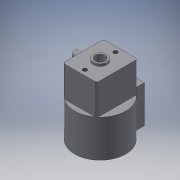
# Autodesk Inventor part: Motor-Body
Saved by Autodesk Inventor 2019 (Build 230136000, 136)
## iProperties
Created: 2021-01-03
Part Number: Motor-Body
Material: Generic
Document SubType Name: Modeling
Designer: Sam
Density: 1 g/cm^3
Appearance: Default
Author: Sam
Autodesk Inventor part; units mm, degrees
ref_plane "YZ Plane" through (0, 0, 0) normal (1, 0, 0) x (0, 1, 0)
ref_plane "XZ Plane" through (0, 0, 0) normal (0, 1, 0) x (-1, 0, 0)
ref_plane "XY Plane" through (0, 0, 0) normal (0, 0, 1) x (1, 0, 0)
sketch "Sketch1" plane through (0, 0, 0) normal (0, 1, 0) x (-1, 0, 0)
  circle A0 centre (0, 0) radius 7.5
  line L0 (-3, -7.5) -> (7, -7.5)
  line L1 (7, -7.5) -> (7, -10)
  line L2 (7, -10) -> (-3, -10)
  line L3 (-3, -10) -> (-3, -7.5)
  circle A1 centre (0, 0) radius 1.5
  dimension "d0" = 15
  dimension "d1" = 3
  dimension "d2" = 10
  dimension "d4" = 10
  dimension "d15" = 3
  constraints: 8 end point, 2 centre point, 2 coincident, 2 parallel, 1 horizontal, 1 perpendicular, 1 tangent
  measures "d0" diameter of A0
  measures "d1" distance from line of point (0, 0) L3
  measures "d2" distance of L1.end L2.end
  measures "d4" distance from line of L2 point (0, 0)
  measures "d15" diameter of A1
extrude "Extrusion3" add sketch "Sketch1" along normal blind 20
sketch "Sketch3" plane through (0, 20, 0) normal (0, 1, 0) x (1, 0, 0)
  line L0 (5, -6) -> (-5, -6)
  line L1 (-5, -6) -> (-5, 6)
  line L2 (-5, 6) -> (5, 6)
  line L3 (5, 6) -> (5, -6)
  line L4 (15, -15) -> (-15, -15)
  line L5 (-15, -15) -> (-15, 15)
  line L6 (-15, 15) -> (15, 15)
  line L7 (15, 15) -> (15, -15)
  point P0 (0, 0)
  point P1 (0, -6)
  point P2 (-5, 0)
  dimension "d18" = 10
  dimension "d19" = 12
  dimension "d20" = 30
  dimension "d21" = 30
  dimension "d22" = 15
  dimension "d23" = 15
  constraints: 16 end point, 4 parallel, 2 horizontal, 2 midpoint, 2 perpendicular, 1 horizontal alignment, 1 vertical alignment
  measures "d18" distance of L0.start L0.end
  measures "d19" distance of L0.end L1.end
  measures "d20" distance of L4.start L4.end
  measures "d21" distance of L6.end L4.start
  measures "d22" distance from line of point (0, 0) L4
  measures "d23" distance from line of point (0, 0) L7
extrude "Extrusion4" cut sketch "Sketch3" against normal blind 9
sketch "Sketch4" plane through (-7, 0, -10) normal (-1, 0, 0) x (0, 0, 1)
  circle A0 centre (1.3, 9.5) radius 1
  circle A1 centre (1.3, 7) radius 1
  circle A2 centre (1.3, 4.5) radius 1
  circle A3 centre (1.3, 2) radius 1
  line L0 (2.5, 0) -> (17.5, 0) projected
  line L1 (0, 0) -> (0, 11) projected
  point P0 (10, 0)
  dimension "d26" = 2
  dimension "d27" = 2.5
  dimension "d28" = 2.5
  dimension "d29" = 2.5
  dimension "d30" = 2
  dimension "d31" = 1.3
  constraints: 4 centre point, 3 equal radius, 3 vertical alignment
  measures "d26" diameter of A0
  measures "d27" distance of A1.centre A0.centre
  measures "d28" distance of A2.centre A1.centre
  measures "d29" distance of A2.centre A3.centre
  measures "d30" distance from line of L0 A3.centre
  measures "d31" distance from line of L1 A3.centre
extrude "Extrusion5" add sketch "Sketch4" along normal blind 9
sketch "Sketch5" plane through (0, 20, 0) normal (0, 1, 0) x (1, 0, 0)
  point P0 (0, 0)
  point P1 (0, -4.5)
  point P2 (0, 4.5)
  dimension "d34" = 9
  dimension "d35" = 4.5
  constraints: 2 vertical alignment
  measures "d34" distance of point (0, 4.5) point (0, -4.5)
  measures "d35" distance of point (0, 0) point (0, -4.5)
hole "Hole1" at (0, 20, 4.5) at (0, 20, -4.5) direction (0, -1, 0) diameter 1.221 depth 5.3 tip angle 118 thread size "M1.6x0.35" class "6H" standard "ISO Metric profile"
sketch "Sketch6" plane through (0, 0, 0) normal (0, -1, 0) x (1, 0, 0)
  circle A0 centre (0, 0) radius 3
  circle A1 centre (0, 0) radius 1.5 projected
  dimension "d43" = 6
  constraints: 1 centre point, 1 coincident
  measures "d43" diameter of A0
extrude "Extrusion6" add sketch "Sketch6" along normal blind 1
sketch "Sketch7" plane through (0, 20, 0) normal (0, 1, 0) x (1, 0, 0)
  circle A0 centre (0, 0) radius 1.5 projected
  circle A1 centre (0, 0) radius 2
  dimension "d46" = 4
  constraints: 1 centre point, 1 coincident
  measures "d46" diameter of A1
extrude "Extrusion7" add sketch "Sketch7" along normal blind 0.7
body "Solid1"
body "Solid2"
